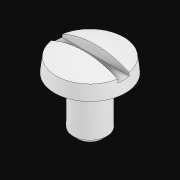
# Autodesk Inventor part: Screw 8-32 Nylon 1.250
Saved by Autodesk Inventor 2021 (Build 250183000, 183)
## iProperties
Created: 2020-07-03
Part Number: Screw 8-32 Nylon 1.250
Material: White
Document SubType Name: Modeling
Designer: yuany
Density: 1 g/cm^3
Appearance: Default
Author: yuany
Autodesk Inventor part; units mm, degrees
ref_plane "YZ Plane" through (0, 0, 0) normal (1, 0, 0) x (0, 1, 0)
ref_plane "XZ Plane" through (0, 0, 0) normal (0, 1, 0) x (-1, 0, 0)
ref_plane "XY Plane" through (0, 0, 0) normal (0, 0, 1) x (1, 0, 0)
sketch "Sketch1" plane through (0, 0, 0) normal (0, 1, 0) x (-1, 0, 0)
  circle A0 centre (0, 0) radius 2.0828
  dimension "d4" = 4.1656
  constraints: 1 centre point, 1 coincident
  measures "d4" diameter of A0
extrude "Body" add sketch "Sketch1" along normal blind 6.35
sketch "Sketch2" plane through (0, 0, 0) normal (1, 0, 0) x (0, 1, 0)
  line L0 (6.35, -2.0828) -> (6.35, 2.0828) projected
  line L1 (6.35, 0) -> (6.35, -4.3688)
  line L2 (8.0772, 0) -> (6.35, 0)
  line L3 (8.0772, 0) -> (8.0772, -4.1656)
  arc A0 (8.0772, -4.1656) -> (9.0169, 0) centre (-0.6859, 0) ccw
  line L4 (6.35, -4.3688) -> (8.0772, -4.1656)
  line L5 (8.0772, 0) -> (9.0169, 0)
  point P0 (0, 0)
  dimension "d5" = 4.3688
  dimension "d13" = 1.7272
  dimension "d57" = 4.1656
  dimension "d58" = 9.7028
  dimension "d59" = 0
  constraints: 10 end point, 2 horizontal, 2 point on circle, 2 point on line, 1 centre point, 1 midpoint, 1 vertical
  measures "d5" distance of L1.start L1.end
  measures "d13" distance of L2.start L1.start
  measures "d57" distance of L2.start L3.end
  measures "d58" radius of A0
  measures "d59" distance from line of L2 A0.centre
revolve "Head" add sketch "Sketch2" angle 360 about axis through (0, 8.0772, 0) along (0, -1, 0)
sketch "Sketch5" plane through (0, 0, 0) normal (1, 0, 0) x (0, 1, 0)
  line L0 (0, -2.0828) -> (6.35, -2.0828) projected
  line L1 (6.35, 4.3688) -> (6.35, -4.3688) projected
  line L2 (6.35, -2.0828) -> (6.35, 2.0828) projected
  line L3 (0.0745, -2.0828) -> (-0.2261, -2.6035)
  line L4 (-0.2261, -2.6035) -> (-0.3253, -2.6035)
  line L5 (-0.3253, -2.6035) -> (-0.626, -2.0828)
  line L6 (0.0686, -2.6035) -> (-0.7252, -2.6035) construction
  line L7 (-0.626, -2.0828) -> (0.0745, -2.0828)
  line L8 (0, -2.0828) -> (6.35, -2.0828) projected
  point P0 (0, 0)
  dimension "d31" = 30
  dimension "d32" = 60
  dimension "a" = 0.0992
  dimension "d46" = 0.7937
  dimension "d54" = 0.0686
  dimension "d55" = 0.5207
  dimension "d56" = 0.0992
  constraints: 10 end point, 2 collinear, 2 point on line, 1 horizontal, 1 perpendicular
  measures "d31" angle of L1 L3
  measures "d32" angle of L3 L5
  measures "a" distance of L3.end L4.end
  measures "d46" distance of L6.start L6.end
  measures "d54" horizontal distance of L6.start L8.start
  measures "d55" distance between parallel lines of L4 L7
  measures "d56" horizontal distance of L5.end L6.end
feature "Thread" [suppressed]
sketch "Sketch6" plane through (0, 0, 0) normal (0, 0, 1) x (1, 0, 0)
  line L0 (0, 0) -> (-1.4859, 0)
  line L1 (2.0828, 0) -> (-2.0828, 0) projected
  line L2 (-1.4859, 0) -> (-2.4948, 1.0089)
  line L3 (-2.4948, 1.0089) -> (-2.9651, -1.2188)
  line L4 (-2.9651, -1.2188) -> (-1.4859, -1.2188)
  line L5 (-2.0828, 0) -> (-2.0828, 6.35) projected
  line L6 (-1.4859, -1.2188) -> (-1.4859, 0)
  line L7 (0, -11.5371) -> (0, 60.6907) projected
  point P0 (-2.0828, 0.5969)
  dimension "d49" = 1.4859
  dimension "d50" = 135
  constraints: 10 end point, 1 perpendicular, 1 point on line, 1 vertical
  measures "d49" distance from line of L0.start L6
  measures "d50" angle of L2 L6
revolve "Tapered End" cut sketch "Sketch6" angle 360 about axis through (0, -10, 0) along (0, 1, 0)
sketch "Sketch7" plane through (0, 0, 0) normal (1, 0, 0) x (0, 1, 0)
  line L0 (6.35, 4.3688) -> (6.35, -4.3688) projected
  line L1 (7.6962, 0.6985) -> (7.6962, -0.6985)
  line L2 (7.6962, 0.6985) -> (9.7028, 0.6985)
  line L3 (9.7028, 0.6985) -> (9.7028, -0.6985)
  line L4 (9.7028, -0.6985) -> (7.6962, -0.6985)
  point P0 (0, 0)
  dimension "d61" = 1.397
  dimension "d62" = 0.6985
  dimension "d65" = 7.6962
  dimension "d66" = 2.0066
  constraints: 8 end point, 1 horizontal, 1 parallel, 1 perpendicular, 1 vertical
  measures "d61" distance of L2.end L3.end
  measures "d62" distance from line of L2 point (0, 0)
  measures "d65" distance from line of point (0, 0) L1
  measures "d66" distance of L1.start L2.end
extrude "Flathead" cut sketch "Sketch7" against normal mid plane 12.7
equation "\"d56\" = a"
body "Solid1"
